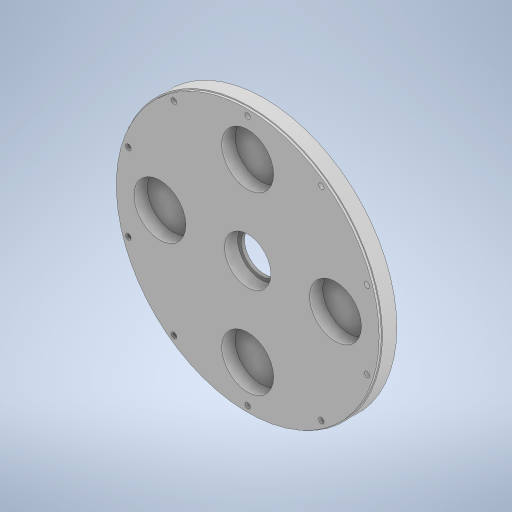
# Autodesk Inventor part: Tampa_Superior
Saved by Autodesk Inventor 2024.2 (Build 282272000, 272)
## iProperties
Created: 2024-04-11
Part Number: Tampa_Superior
Material: Generic
Document SubType Name: Modeling
Designer: 062210029
Density: 1 g/cm^3
Appearance: Default
Author: 062210029
Autodesk Inventor part; units mm, degrees
ref_plane "YZ Plane" through (0, 0, 0) normal (1, 0, 0) x (0, 1, 0)
ref_plane "XZ Plane" through (0, 0, 0) normal (0, 1, 0) x (-1, 0, 0)
ref_plane "XY Plane" through (0, 0, 0) normal (0, 0, 1) x (1, 0, 0)
sketch "Sketch1" plane through (0, 0, 0) normal (0, 0, 1) x (1, 0, 0)
  circle A0 centre (0, 0) radius 120
  circle A1 centre (0, 0) radius 18
  dimension "d0" = 240
  dimension "d1" = 36
  constraints: 2 centre point, 2 coincident
  measures "d0" diameter of A0
  measures "d1" diameter of A1
extrude "Extrusion1" add sketch "Sketch1" along normal blind 15
sketch "Sketch2" plane through (0, 0, 15) normal (0, 0, 1) x (1, 0, 0)
  circle A0 centre (79.5, 0) radius 23.5
  circle A1 centre (0, 79.5) radius 23.5
  circle A2 centre (-79.5, 0) radius 23.5
  circle A3 centre (0, -79.5) radius 23.5
  point P0 (0, 0)
  dimension "d5" = 47
  dimension "d7" = 47
  dimension "d8" = 47
  dimension "d9" = 47
  constraints: 4 centre point
  measures "d5" diameter of A0
  measures "d7" diameter of A1
  measures "d8" diameter of A2
  measures "d9" diameter of A3
extrude "Extrusion2" cut sketch "Sketch2" against normal blind 12
sketch "Sketch3" plane through (0, 0, 15) normal (0, 0, 1) x (1, 0, 0)
  circle A0 centre (0, 0) radius 21
  dimension "d12" = 42
  constraints: 1 centre point, 1 coincident
  measures "d12" diameter of A0
extrude "Extrusion3" cut sketch "Sketch3" against normal blind 12
sketch "Sketch4" plane through (0, 0, 15) normal (0, 0, 1) x (1, 0, 0)
  circle A0 centre (0, 0) radius 18 projected
  circle A1 centre (0, 0) radius 119
  circle A2 centre (0, 0) radius 120
  dimension "d15" = 238
  dimension "d16" = 240
  constraints: 2 centre point, 2 coincident
  measures "d15" diameter of A1
  measures "d16" diameter of A2
extrude "Extrusion4" cut sketch "Sketch4" against normal blind 2 contours A2
sketch "Sketch5" plane through (0, 0, 15) normal (0, 0, 1) x (1, 0, 0)
  circle A0 centre (0, 0) radius 21 projected
  line L0 (0, 0) -> (0, 113.556) construction
  circle A1 centre (0, 113.556) radius 2.5
  circle A2 centre (0, 0) radius 18 projected
  circle A3 centre (0, 0) radius 113.556
  circle A4 centre (-66.7465, 91.8687) radius 2.5
  circle A5 centre (-107.9982, 35.0907) radius 2.5
  circle A6 centre (-107.9982, -35.0907) radius 2.5
  circle A7 centre (-66.7465, -91.8687) radius 2.5
  circle A8 centre (0, -113.556) radius 2.5
  circle A9 centre (66.7465, -91.8687) radius 2.5
  circle A10 centre (107.9982, -35.0907) radius 2.5
  circle A11 centre (107.9982, 35.0907) radius 2.5
  circle A12 centre (66.7465, 91.8687) radius 2.5
  dimension "d19" = 113.556
  dimension "d20" = 5
  dimension "d24" = 360
  constraints: 10 centre point, 2 coincident, 2 end point, 1 vertical, 1 vertical alignment, 23 other
  measures "d19" distance of L0.start L0.end
  measures "d20" diameter of A1
extrude "Extrusion5" cut sketch "Sketch5" against normal blind 15 contours A1 A3 | A3 A1 | A4 A3 | A3 A4 | A12 A3 | A3 A12 | A5 A3 | A3 A5 | A11 A3 | A3 A11 | A6 A3 | A3 A6 | A10 A3 | A3 A10 | A7 A3 | A3 A7 | A9 A3 | A3 A9 | A8 A3 | A3 A8
sketch "Sketch7" plane through (0, 0, 0) normal (0, 0, -1) x (-1, 0, 0)
  circle A0 centre (0, 113.556) radius 2.5 projected
  circle A1 centre (0, 113.556) radius 6.12
  circle A2 centre (0, 0) radius 113.556 construction
  circle A3 centre (0, 0) radius 113.556 construction
  circle A4 centre (-66.7465, 91.8687) radius 6.12
  circle A5 centre (0, 0) radius 113.556 construction
  circle A6 centre (-107.9982, 35.0907) radius 6.12
  circle A7 centre (0, 0) radius 113.556 construction
  circle A8 centre (-107.9982, -35.0907) radius 6.12
  circle A9 centre (0, 0) radius 113.556 construction
  circle A10 centre (-66.7465, -91.8687) radius 6.12
  circle A11 centre (0, 0) radius 113.556 construction
  circle A12 centre (0, -113.556) radius 6.12
  circle A13 centre (0, 0) radius 113.556 construction
  circle A14 centre (66.7465, -91.8687) radius 6.12
  circle A15 centre (0, 0) radius 113.556 construction
  circle A16 centre (107.9982, -35.0907) radius 6.12
  circle A17 centre (0, 0) radius 113.556 construction
  circle A18 centre (107.9982, 35.0907) radius 6.12
  circle A19 centre (0, 0) radius 113.556 construction
  circle A20 centre (66.7465, 91.8687) radius 6.12
  dimension "d28" = 12.24
  dimension "d31" = 360
  constraints: 10 centre point, 4 coincident, 2 vertical alignment, 67 other
  measures "d28" diameter of A1
extrude "Extrusion6" cut sketch "Sketch7" against normal blind 2 contours A0 | A1 | A4 | A6 | A8 | A10 | A12 | A14 | A16 | A18 | A20
body "Solid1"
